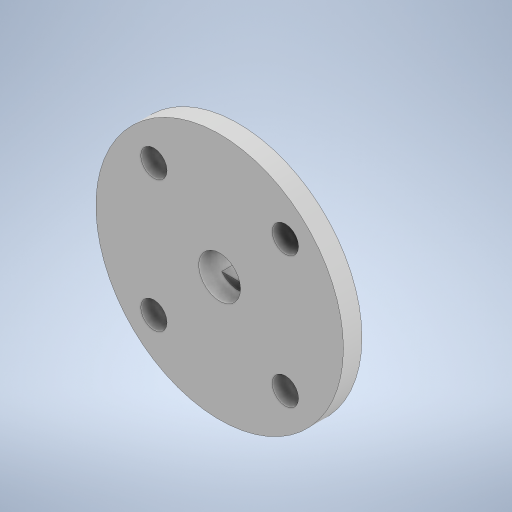
# Autodesk Inventor part: Wheel_2D_Eje
Saved by Autodesk Inventor 2023 (Build 270158000, 158)
## iProperties
Created: 2024-08-05
Part Number: Wheel_2D_Eje
Material: Generic
Document SubType Name: Modeling
Designer: LEGION
Density: 1 g/cm^3
Appearance: Default
Author: LEGION
Autodesk Inventor part; units mm, degrees
ref_plane "YZ Plane" through (0, 0, 0) normal (1, 0, 0) x (0, 1, 0)
ref_plane "XZ Plane" through (0, 0, 0) normal (0, 1, 0) x (-1, 0, 0)
ref_plane "XY Plane" through (0, 0, 0) normal (0, 0, 1) x (1, 0, 0)
sketch "Sketch1" plane through (0, 0, 0) normal (0, 0, 1) x (1, 0, 0)
  circle A0 centre (0, 0) radius 5
  circle A1 centre (0, 0) radius 2.7
  line L0 (-2.1372, 1.65) -> (2.1372, 1.65)
  line L1 (2.1372, -1.65) -> (-2.1372, -1.65)
  line L2 (2, 0.4) -> (5, 0.4)
  line L3 (5, 0.4) -> (5, -0.4)
  line L4 (5, -0.4) -> (2, -0.4)
  line L5 (2, -0.4) -> (2, 0.4)
  point P0 (4.984, -0.4)
  point P1 (2.6702, -0.4)
  point P2 (2.6702, 0.4)
  point P3 (4.984, 0.4)
  dimension "d0" = 5.4
  dimension "d1" = 3.3
  dimension "d2" = 1.65
  dimension "d3" = 10
  dimension "d4" = 0.4
  dimension "d5" = 0.4
  dimension "d6" = 2
  constraints: 12 end point, 4 point on circle, 3 parallel, 2 centre point, 2 coincident, 2 horizontal, 1 perpendicular, 1 tangent
  measures "d0" diameter of A1
  measures "d1" distance between parallel lines of L1 L0
  measures "d2" distance from line of point (0, 0) L1
  measures "d3" diameter of A0
  measures "d4" distance from line of point (0, 0) L4
  measures "d5" distance from line of point (0, 0) L2
  measures "d6" distance from line of point (0, 0) L5
extrude "Extrusion1" add sketch "Sketch1" along normal blind 7 contours A0 L4 A1 L2 | L2 A1 L4 A0 | L0 A1 | A1 L1
sketch "Sketch2" plane through (0, 0, 7) normal (0, 0, 1) x (1, 0, 0)
  circle A0 centre (0, 0) radius 16
  circle A1 centre (-8.5, 8.5) radius 1.7
  circle A2 centre (8.5, 8.5) radius 1.7
  circle A3 centre (-8.5, -8.5) radius 1.7
  circle A4 centre (8.5, -8.5) radius 1.7
  line L0 (8.5, 8.5) -> (8.5, -8.5)
  line L1 (8.5, -8.5) -> (-8.5, -8.5)
  line L2 (-8.5, -8.5) -> (-8.5, 8.5)
  line L3 (-8.5, 8.5) -> (8.5, 8.5)
  circle A5 centre (0, 0) radius 2.7
  dimension "d9" = 17
  dimension "d10" = 17
  dimension "d11" = 8.5
  dimension "d12" = 8.5
  dimension "d13" = 3.4
  dimension "d14" = 3.4
  dimension "d15" = 3.4
  dimension "d16" = 3.4
  dimension "d17" = 32
  dimension "d18" = 5.4
  constraints: 8 end point, 6 centre point, 3 perpendicular, 2 coincident, 1 vertical
  measures "d9" distance of L0.start L0.end
  measures "d10" distance of L2.end L0.start
  measures "d11" distance from line of L3 point (0, 0)
  measures "d12" distance from line of L0 point (0, 0)
  measures "d13" diameter of A2
  measures "d14" diameter of A1
  measures "d15" diameter of A4
  measures "d16" diameter of A3
  measures "d17" diameter of A0
  measures "d18" diameter of A5
extrude "Extrusion2" add sketch "Sketch2" along normal blind 2.4 contours A0 | L3 A2 L0 A4 L1 A3 L2 A1
sketch "Sketch6" plane through (0, 0, 0) normal (0, 0, -1) x (-1, 0, 0)
  line L0 (-4.9, -1.65) -> (4.9, -1.65)
  line L1 (4.9, -1.65) -> (4.9, -8.75)
  line L2 (4.9, -8.75) -> (-4.9, -8.75)
  line L3 (-4.9, -8.75) -> (-4.9, -1.65)
  line L4 (-2.9, -2.85) -> (2.9, -2.85)
  line L5 (2.9, -2.85) -> (2.9, -5.75)
  line L6 (2.9, -5.75) -> (-2.9, -5.75)
  line L7 (-2.9, -5.75) -> (-2.9, -2.85)
  arc A0 (-2.1372, 1.65) -> (-2.1372, -1.65) centre (0, 0) ccw projected
  line L8 (2.1372, 1.65) -> (-2.1372, 1.65) projected
  arc A1 (2.1372, -1.65) -> (2.1372, 1.65) centre (0, 0) ccw projected
  line L9 (-2.1372, -1.65) -> (2.1372, -1.65) projected
  circle A2 centre (0, 0) radius 5 projected
  line L10 (4.9, -1.65) -> (3.4, -1.65)
  line L11 (3.4, -1.65) -> (3.4, 0)
  line L12 (3.4, 0) -> (4.9, 0)
  line L13 (4.9, 0) -> (4.9, -1.65)
  line L14 (-4.9, -1.65) -> (-3.4, -1.65)
  line L15 (-3.4, -1.65) -> (-3.4, 0)
  line L16 (-3.4, 0) -> (-4.9, 0)
  line L17 (-4.9, 0) -> (-4.9, -1.65)
  point P0 (-4.9, -0.995)
  point P1 (4.9, -0.995)
  point P2 (2.9, -4.0731)
  point P3 (-2.9, -4.0731)
  dimension "d37" = 1.2
  dimension "d38" = 5.8
  dimension "d39" = 0
  dimension "d40" = 2.9
  dimension "d41" = 3
  dimension "d42" = 2.9
  dimension "d43" = 2
  dimension "d44" = 2
  dimension "d45" = 1.5
  dimension "d46" = 1.5
  constraints: 32 end point, 8 parallel, 4 horizontal, 4 perpendicular, 2 horizontal alignment
  measures "d37" distance between parallel lines of L0 L4
  measures "d38" distance of L4.start L4.end
  measures "d39" distance between parallel lines of L9 L0
  measures "d40" distance between parallel lines of L4 L6
  measures "d41" distance between parallel lines of L2 L6
  measures "d42" distance from line of L5 point (0, 0)
  measures "d43" distance between parallel lines of L1 L5
  measures "d44" distance between parallel lines of L7 L3
  measures "d45" distance of L11.end L12.end
  measures "d46" distance of L15.end L16.end
extrude "Extrusion6" add sketch "Sketch6" against normal blind 7 contours A2 L7 L6 L5 L0 L1 L2 L3 | L0 L17 A2 | A2 L13 L0
sketch "Sketch7" plane through (0, 0, 0) normal (0, 0, -1) x (-1, 0, 0)
  line L0 (-2.9, -5.75) -> (-2.9, -4.0731) projected
  line L1 (-2.9, -5.75) -> (2.9, -5.75)
  line L2 (2.9, -5.75) -> (2.9, -2.85)
  line L3 (2.9, -2.85) -> (-2.9, -2.85)
  line L4 (-2.9, -2.85) -> (-2.9, -5.75)
  line L5 (2.9, -4.0731) -> (2.9, -5.75) projected
  point P0 (0, 0)
  dimension "d49" = 2.9
  constraints: 8 end point, 2 parallel, 1 collinear, 1 horizontal, 1 perpendicular
  measures "d49" distance between parallel lines of L1 L3
extrude "Extrusion7" cut sketch "Sketch7" against normal blind 7
sketch "Sketch8" plane through (-4.9, -8.75, 0) normal (0, -1, 0) x (1, 0, 0)
  circle A0 centre (4.9, 3.5) radius 1.7
  line L0 (9.8, 0) -> (0, 0) projected
  point P0 (4.9, 0)
  point P1 (4.9, 0)
  dimension "d52" = 3.4
  dimension "d53" = 3.5
  constraints: 1 centre point, 1 midpoint, 1 vertical alignment
  measures "d52" diameter of A0
  measures "d53" distance from line of L0 A0.centre
extrude "Extrusion8" cut sketch "Sketch8" against normal blind 8
fillet "Fillet1" radius 1.5 6 edges at (-4.9, -8.75, 3.5) (4.9, -8.75, 3.5) (-4.9, -4.8725, 7) (0, 5, 7) (4.9, -4.8725, 7) (0, -8.75, 7)
equation "\"d2\" = 0.5 * d1"
equation "\"d4\" = d5"
equation "\"d9\" = d10"
equation "\"d11\" = 0.5 * d9"
equation "\"d12\" = d11"
equation "\"d42\" = 0.5 * d38"
body "Solid1"
